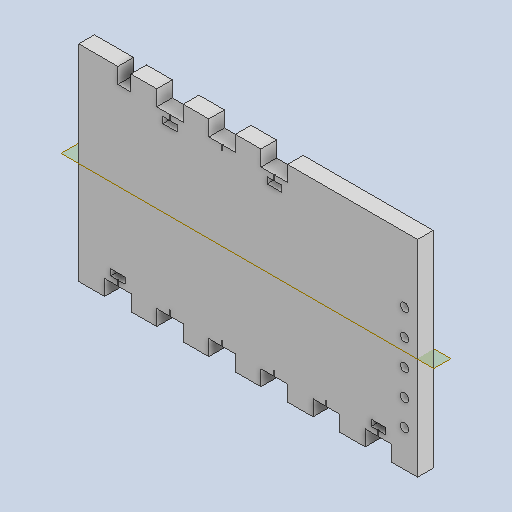
# Autodesk Inventor part: 00_Baseplate_Simmo_side2_v2
Saved by Autodesk Inventor 2022 (Build 260153000, 153)
## iProperties
Created: 2022-08-03
Part Number: 00_Baseplate_Simmo_side2_v2
Material: Generic
Document SubType Name: Modeling
Designer: wanghaoran
Density: 1 g/cm^3
Appearance: Default
Author: wanghaoran
Autodesk Inventor part; units mm, degrees
ref_plane "YZ Plane" through (0, 0, 0) normal (1, 0, 0) x (0, 1, 0)
ref_plane "XZ Plane" through (0, 0, 0) normal (0, 1, 0) x (-1, 0, 0)
ref_plane "XY Plane" through (0, 0, 0) normal (0, 0, 1) x (1, 0, 0)
sketch "Sketch1" plane through (0, 0, 0) normal (0, 0, 1) x (1, 0, 0)
  line L0 (-20, 6) -> (-10, 6) projected
  line L1 (-70, 0) -> (-70, 6) projected
  line L2 (-75, 6) -> (-70, 6) projected
  line L3 (-75, 0) -> (-75, 6) projected
  line L4 (-75, 0) -> (-70, 0) projected
  line L5 (40, -67) -> (40, -9) projected
  line L6 (40, 6) -> (-90, 6)
  line L7 (-90, 6) -> (-90, -73)
  line L8 (-90, -73) -> (40, -73)
  line L9 (40, -73) -> (40, 6)
  point P0 (0, 0)
  point P1 (40, -67)
  point P2 (40, -9)
  point P3 (-90, 0)
  point P4 (-75, 6)
  dimension "d0" = 79
  constraints: 8 end point, 2 parallel, 1 horizontal, 1 perpendicular, 1 point on line
  measures "d0" distance of L7.end L6.end
extrude "Extrusion1" add sketch "Sketch1" along normal blind 6 contours L0 L6 L9 L5 L8 L7 L3 L4 L1
ref_plane "Work Plane1" through (-90, -33.5, 0) normal (0, -1, 0) x (1, 0, 0)
sketch "Sketch2" plane through (0, 0, 6) normal (0, 0, 1) x (1, 0, 0)
  line L0 (-60, 6) -> (-60, 0) projected
  line L1 (-60, 0) -> (-50, 0) projected
  line L2 (-50, 0) -> (-50, 6) projected
  line L3 (-40, 0) -> (-30, 0) projected
  line L4 (-30, 0) -> (-30, 6) projected
  line L5 (-40, 6) -> (-40, 0) projected
  line L6 (-20, 0) -> (-10, 0) projected
  line L7 (-20, 6) -> (-20, 0) projected
  line L8 (-10, 0) -> (-10, 6) projected
  line L9 (40, 6) -> (-70, 6) projected
  line L10 (-50, 6) -> (-49.9, 6)
  line L11 (-49.9, 6) -> (-49.9, 0)
  line L12 (-49.9, 0) -> (-50, 0)
  line L13 (-50, 0) -> (-50, 6)
  line L14 (-60, 6) -> (-60.1, 6)
  line L15 (-60.1, 6) -> (-60.1, 0)
  line L16 (-60.1, 0) -> (-60, 0)
  line L17 (-60, 0) -> (-60, 6)
  point P0 (0, 0)
  dimension "d5" = 0.1
  dimension "d6" = 6
  dimension "d7" = 0.1
  dimension "d8" = 6
  constraints: 16 end point, 4 parallel, 2 horizontal, 2 perpendicular
  measures "d5" distance of L11.end L12.end
  measures "d6" distance of L10.end L11.end
  measures "d7" distance of L16.end L15.end
  measures "d8" distance of L15.end L14.end
extrude "Extrusion2" cut sketch "Sketch2" against normal blind 6 contours L9 L2 L1 L0 | L0 L16 L15 L9 | L9 L11 L12 L2
pattern_linear "Rectangular Pattern1" count 3 spacing 20 along (1, 0, 0) of "Extrusion2"
sketch "Sketch3" plane through (0, 0, 6) normal (0, 0, 1) x (1, 0, 0)
  circle A0 centre (35, -59) radius 1.4 projected
  circle A1 centre (35, -39) radius 1.4 projected
  circle A2 centre (35, -29) radius 1.4 projected
  circle A3 centre (35, -49) radius 1.4 projected
  circle A4 centre (35, -19) radius 1.4 projected
  point P0 (0, 0)
sketch "Sketch4" plane through (0, 0, 6) normal (0, 0, 1) x (1, 0, 0)
  line L0 (-60.1, 0) -> (-60.1, 6) projected
  line L1 (-60, 0) -> (-50, 0) projected
  line L2 (-49.9, 6) -> (-49.9, 0) projected
  line L3 (-49.9, 0) -> (-60.1, 0) projected
  line L4 (66, -33.5) -> (-116, -33.5) projected
  line L5 (-60.1, -67) -> (-60.1, -73)
  line L6 (-49.9, -73) -> (-49.9, -67)
  line L7 (-49.9, -67) -> (-60.1, -67)
  line L8 (-90, -73) -> (40, -73) projected
  line L9 (-69.9, -73) -> (-69.9, -67)
  line L10 (-69.9, -67) -> (-80.1, -67)
  line L11 (-80.1, -67) -> (-80.1, -73)
  line L12 (-29.9, -73) -> (-29.9, -67)
  line L13 (-29.9, -67) -> (-40.1, -67)
  line L14 (-40.1, -67) -> (-40.1, -73)
  line L15 (-49.9, -73) -> (-49.9, -67)
  line L16 (-49.9, -67) -> (-60.1, -67)
  line L17 (-60.1, -67) -> (-60.1, -73)
  line L18 (-9.9, -73) -> (-9.9, -67)
  line L19 (-9.9, -67) -> (-20.1, -67)
  line L20 (-20.1, -67) -> (-20.1, -73)
  line L21 (-29.9, -73) -> (-29.9, -67)
  line L22 (-29.9, -67) -> (-40.1, -67)
  line L23 (-40.1, -67) -> (-40.1, -73)
  line L24 (10.1, -73) -> (10.1, -67)
  line L25 (10.1, -67) -> (-0.1, -67)
  line L26 (-0.1, -67) -> (-0.1, -73)
  line L27 (-9.9, -73) -> (-9.9, -67)
  line L28 (-9.9, -67) -> (-20.1, -67)
  line L29 (-20.1, -67) -> (-20.1, -73)
  line L30 (30.1, -73) -> (30.1, -67)
  line L31 (30.1, -67) -> (19.9, -67)
  line L32 (19.9, -67) -> (19.9, -73)
  line L33 (10.1, -73) -> (10.1, -67)
  line L34 (10.1, -67) -> (-0.1, -67)
  line L35 (-0.1, -67) -> (-0.1, -73)
  point P0 (0, 0)
  dimension "d16" = 20
  dimension "d19" = 20
  constraints: 60 end point, 4 symmetric about line, 2 collinear, 2 horizontal, 61 other
  measures "d16" distance of L6.start L9.start
  measures "d19" distance of L6.start L12.start
extrude "Extrusion4" cut sketch "Sketch4" against normal blind 6
hole "Hole1" at (35, -59, 6) at (35, -49, 6) at (35, -39, 6) at (35, -29, 6) at (35, -19, 6) direction (0, 0, -1) diameter 3.2 depth 6
sketch "Sketch5" plane through (0, 0, 6) normal (0, 0, 1) x (1, 0, 0)
  line L0 (-9.9, 0) -> (-20.1, 0) projected
  line L1 (-15, 0) -> (-14.8, 0)
  line L2 (-14.8, 0) -> (-14.8, -2)
  line L3 (-14.8, -2) -> (-15, -2)
  line L4 (-15, -2) -> (-15, 0)
  line L5 (-15, 0) -> (-15.2, 0)
  line L6 (-15.2, 0) -> (-15.2, -2)
  line L7 (-15.2, -2) -> (-15, -2)
  line L8 (-15, -2) -> (-15, 0)
  point P0 (0, 0)
  dimension "d31" = 0.2
  dimension "d32" = 2
  dimension "d33" = 0.2
  dimension "d34" = 2
  constraints: 16 end point, 4 parallel, 2 horizontal, 2 perpendicular, 1 midpoint
  measures "d31" distance of L2.end L3.end
  measures "d32" distance of L1.end L2.end
  measures "d33" distance of L7.end L6.end
  measures "d34" distance of L6.end L5.end
extrude "Extrusion5" cut sketch "Sketch5" against normal blind 0.2
pattern_linear "Rectangular Pattern2" count 3 spacing 20 along (-1, 0, 0) of "Extrusion5"
sketch "Sketch6" plane through (0, 0, 6) normal (0, 0, 1) x (1, 0, 0)
  line L0 (-69.9, -67) -> (-80.1, -67) projected
  line L1 (-75, -67) -> (-74.8, -67)
  line L2 (-74.8, -67) -> (-74.8, -65)
  line L3 (-74.8, -65) -> (-75, -65)
  line L4 (-75, -65) -> (-75, -67)
  line L5 (-75, -67) -> (-75.2, -67)
  line L6 (-75.2, -67) -> (-75.2, -65)
  line L7 (-75.2, -65) -> (-75, -65)
  line L8 (-75, -65) -> (-75, -67)
  point P0 (0, 0)
  dimension "d40" = 0.2
  dimension "d41" = 2
  dimension "d42" = 0.2
  dimension "d43" = 2
  constraints: 16 end point, 4 parallel, 2 horizontal, 2 perpendicular, 1 midpoint
  measures "d40" distance of L3.end L2.end
  measures "d41" distance of L2.end L1.end
  measures "d42" distance of L6.end L7.end
  measures "d43" distance of L5.end L6.end
extrude "Extrusion6" cut sketch "Sketch6" against normal blind 0.2
pattern_linear "Rectangular Pattern3" count 6 spacing 20 along (1, 0, 0) of "Extrusion6"
sketch "Sketch7" plane through (0, 0, 6) normal (0, 0, 1) x (1, 0, 0)
  line L0 (27.75, -65) -> (22.25, -65)
  line L1 (22.25, -65) -> (22.25, -62.6)
  line L2 (22.25, -62.6) -> (27.75, -62.6)
  line L3 (27.75, -62.6) -> (27.75, -65)
  line L4 (10.1, -73) -> (19.9, -73) projected
  line L5 (30.1, -67) -> (30.1, -73) projected
  line L6 (-77.75, -62.6) -> (-72.25, -62.6)
  line L7 (-72.25, -62.6) -> (-72.25, -65)
  line L8 (-72.25, -65) -> (-77.75, -65)
  line L9 (-77.75, -65) -> (-77.75, -62.6)
  line L10 (-12.25, -4.4) -> (-17.75, -4.4)
  line L11 (-17.75, -4.4) -> (-17.75, -2)
  line L12 (-17.75, -2) -> (-12.25, -2)
  line L13 (-12.25, -2) -> (-12.25, -4.4)
  line L14 (-20.1, 6) -> (-29.9, 6) projected
  line L15 (-9.9, 6) -> (-9.9, 0) projected
  line L16 (-52.25, -4.4) -> (-57.75, -4.4)
  line L17 (-57.75, -2) -> (-52.25, -2)
  line L18 (-52.25, -2) -> (-52.25, -4.4)
  line L19 (-57.75, -4.4) -> (-57.75, -2)
  point P0 (0, 0)
  dimension "d49" = 5.5
  dimension "d50" = 2.4
  dimension "d51" = 8
  dimension "d52" = 2.35
  dimension "d55" = 100
  dimension "d60" = 5.5
  dimension "d61" = 2.4
  dimension "d62" = 8
  dimension "d63" = 2.35
  dimension "d66" = 40
  constraints: 32 end point, 4 horizontal, 4 parallel, 2 collinear, 2 perpendicular, 14 other
  measures "d49" distance of L1.end L2.end
  measures "d50" distance of L0.end L1.end
  measures "d51" distance between parallel lines of L4 L0
  measures "d52" distance between parallel lines of L5 L3
  measures "d55" distance of L1.end L6.start
  measures "d60" distance of L11.end L12.end
  measures "d61" distance of L10.end L11.end
  measures "d62" distance between parallel lines of L14 L12
  measures "d63" distance between parallel lines of L15 L13
  measures "d66" distance of L10.start L16.start
extrude "Extrusion7" cut sketch "Sketch7" against normal blind 6
body "Solid1"
